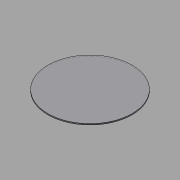
# Autodesk Inventor part: pcb
Saved by Autodesk Inventor 2015 (Build 190159000, 159)
## iProperties
Created: 2016-09-28
Part Number: pcb
Material: PC/ABS Plastic
Document SubType Name: Modeling
Designer: Paulo Loma
Density: 0.357273 g/cm^3
Appearance: Smooth - White
Author: Paulo Loma
Autodesk Inventor part; units mm, degrees
ref_plane "YZ Plane" through (0, 0, 0) normal (1, 0, 0) x (0, 1, 0)
ref_plane "XZ Plane" through (0, 0, 0) normal (0, 1, 0) x (-1, 0, 0)
ref_plane "XY Plane" through (0, 0, 0) normal (0, 0, 1) x (1, 0, 0)
sketch "Sketch1" plane through (0, 0, 0) normal (0, 0, 1) x (1, 0, 0)
  circle A0 centre (-4.4344, 11.349) radius 32.5
  point P0 (0, 0)
  dimension "d0" = 65
  dimension "d0" = 65
  constraints: 1 centre point
  measures "d0" diameter of A0
extrude "Extrusion1" add sketch "Sketch1" along normal blind 1
body "Solid1"
